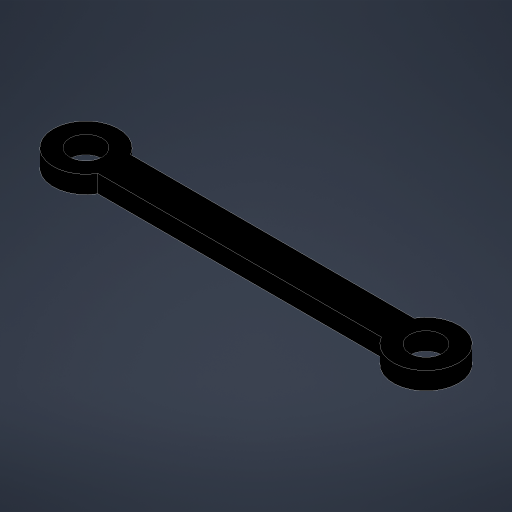
# Autodesk Inventor part: FP V2 Batang Penggerak
Saved by Autodesk Inventor 2023.6 (Build 276521000, 521)
## iProperties
Created: 2026-02-13
Part Number: FP V2 Batang Penggerak
Material: Aluminum 6061
Document SubType Name: Modeling
Designer: user
Density: 2.7 g/cm^3
Appearance: Anodized - Black
Author: user
Autodesk Inventor part; units mm, degrees
ref_plane "YZ Plane" through (0, 0, 0) normal (1, 0, 0) x (0, 1, 0)
ref_plane "XZ Plane" through (0, 0, 0) normal (0, 1, 0) x (-1, 0, 0)
ref_plane "XY Plane" through (0, 0, 0) normal (0, 0, 1) x (1, 0, 0)
sketch "Sketch1" plane through (0, 0, 0) normal (0, 1, 0) x (-1, 0, 0)
  line L0 (0, 0) -> (57, 0)
  line L1 (57, 0) -> (57, 5)
  line L2 (57, 5) -> (0, 5)
  line L3 (0, 5) -> (0, 0)
  circle A0 centre (54.5, 2.5) radius 2.5
  circle A1 centre (2.5, 2.5) radius 2.5
  circle A2 centre (54.5, 2.5) radius 5
  circle A3 centre (2.5, 2.5) radius 5
  line L4 (57, 0) -> (57, 5)
  line L5 (57, 2.5) -> (0, 2.5)
  point P0 (50.1699, 0)
  point P1 (50.1699, 5)
  point P2 (6.8301, 5)
  point P3 (6.8301, 0)
  dimension "d0" = 5
  dimension "d1" = 57
  dimension "d2" = 5
  dimension "d3" = 5
  dimension "d4" = 10
  dimension "d5" = 10
  constraints: 12 end point, 4 centre point, 3 equal length, 2 coincident, 2 midpoint, 2 point on line, 2 tangent, 1 horizontal, 1 perpendicular
  measures "d0" distance between parallel lines of L0 L2
  measures "d1" distance between parallel lines of L3 L1
  measures "d2" diameter of A0
  measures "d3" diameter of A1
  measures "d4" diameter of A2
  measures "d5" diameter of A3
extrude "Extrusion1" add sketch "Sketch1" along normal blind 2.7 contours L3 A1 L0 | L0 A3 L2 L3 | A1 L5 A3 L0 | L3 L2 A1 | A3 L5 A2 L0 | A1 L2 A3 L5 | A2 L5 A0 L0 | L0 L1 L2 A2 | L2 A2 L5 A3 | A0 L1 L0 | A2 L2 A0 L5 | A0 L2 L1
body "Solid1"
